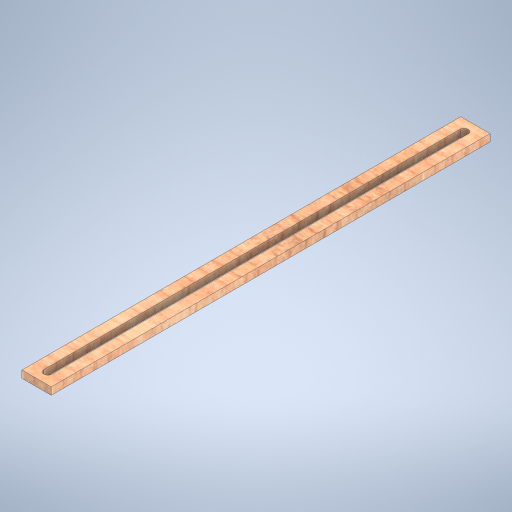
# Autodesk Inventor part: XYarm
Saved by Autodesk Inventor 2023 (Build 270158000, 158)
## iProperties
Created: 2023-10-26
Part Number: XYarm
Material: Wood (Birch)
Document SubType Name: Modeling
Designer: Mustapha
Density: 0.55 g/cm^3
Appearance: Birch - Natural Polished
Mass: 10.1379 g
Surface Area: 125.044 cm^2
Volume: 18.4325 cm^3
Author: Mustapha
Autodesk Inventor part; units mm, degrees
ref_plane "YZ Plane" through (0, 0, 0) normal (1, 0, 0) x (0, 1, 0)
ref_plane "XZ Plane" through (0, 0, 0) normal (0, 1, 0) x (-1, 0, 0)
ref_plane "XY Plane" through (0, 0, 0) normal (0, 0, 1) x (1, 0, 0)
sketch "Sketch1" plane through (0, 0, 0) normal (0, 1, 0) x (-1, 0, 0)
  line L0 (0, 142.25) -> (0, -142.25) construction
  line L1 (2.75, 142.25) -> (2.75, -142.25)
  line L2 (-2.75, -142.25) -> (-2.75, 142.25)
  arc A0 (2.75, 142.25) -> (-2.75, 142.25) centre (0, 142.25) ccw
  arc A1 (-2.75, -142.25) -> (2.75, -142.25) centre (0, -142.25) ccw
  line L3 (-10, -150) -> (10, -150)
  line L4 (10, -150) -> (10, 150)
  line L5 (10, 150) -> (-10, 150)
  line L6 (-10, 150) -> (-10, -150)
  line L7 (-10, -150) -> (10, 150) construction
  line L8 (10, -150) -> (-10, 150) construction
  point P0 (0, 0)
  point P1 (0, -145)
  point P2 (0, 145)
  dimension "d0" = 290
  dimension "d1" = 5.5
  dimension "d2" = 300
  dimension "d3" = 20
  constraints: 20 end point, 6 point on circle, 4 tangent, 3 midpoint, 3 parallel, 2 centre point, 1 horizontal, 1 perpendicular, 1 vertical
  measures "d0" distance of point (0, -145) point (0, 145)
  measures "d1" distance between parallel lines of L2 L1
  measures "d2" distance between parallel lines of L3 L5
  measures "d3" distance between parallel lines of L6 L4
extrude "Extrusion1" add sketch "Sketch1" along normal blind 5
body "Solid1"
